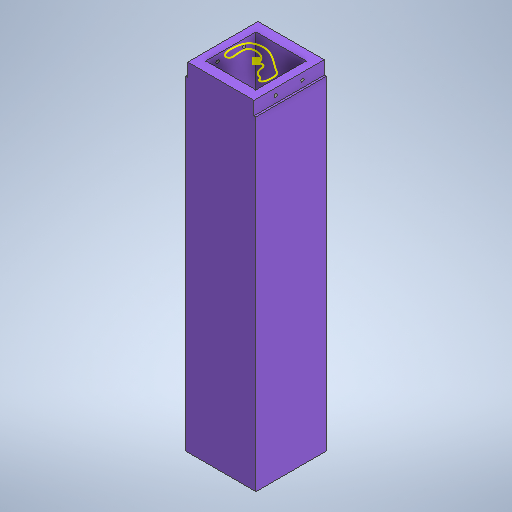
# Autodesk Inventor part: TS_Magazin_int
Saved by Autodesk Inventor 2025.2 (Build 292293000, 293)
## iProperties
Created: 2025-05-27
Part Number: TS_Magazin_int
Material: Generisch
Document SubType Name: Modeling
Designer: tino
Density: 1 g/cm^3
Appearance: Vorgabe
Mass: 3200 g
Surface Area: 1728 cm^2
Volume: 3200 cm^3
Author: tino
Autodesk Inventor part; units mm, degrees
ref_plane "YZ Plane" through (0, 0, 0) normal (1, 0, 0) x (0, 1, 0)
ref_plane "XZ Plane" through (0, 0, 0) normal (0, 1, 0) x (-1, 0, 0)
ref_plane "XY Plane" through (0, 0, 0) normal (0, 0, 1) x (1, 0, 0)
sketch "Skizze1" plane through (0, 0, 0) normal (0, 0, 1) x (1, 0, 0)
  line L0 (-52.5, 52.5) -> (52.5, 52.5)
  line L1 (52.5, 52.5) -> (52.5, -52.5)
  line L2 (52.5, -52.5) -> (-52.5, -52.5)
  line L3 (-52.5, -52.5) -> (-52.5, 52.5)
  line L4 (-52.5, 52.5) -> (52.5, -52.5) construction
  line L5 (52.5, 52.5) -> (-52.5, -52.5) construction
  point P0 (0, 0)
  dimension "d0" = 105
  dimension "d1" = 105
  constraints: 12 end point, 2 midpoint, 2 parallel, 1 horizontal, 1 perpendicular
  measures "d0" distance of L0.start L0.end
  measures "d1" distance of L0.end L1.end
extrude "Extrusion1" add sketch "Skizze1" along normal blind 505
sketch "Skizze2" plane through (0, 0, 505) normal (0, 0, 1) x (1, 0, 0)
  spline S0 degree 3 poles (30.8941, -22.3608) (33.2455, -20.1357) (33.4278, -16.4642) (34.1009, -12.3897) (34.4408, -6.5615) (32.3239, 0.3889) (27.6464, 2.563) (18.7777, 8.3579) (6.0522, 19.3643) (-10.5838, 24.0919) (-22.9306, 22.7109) (-28.1368, 17.5955) (-28.9312, 16.6042) knots 0 0 0 0 0.05535 0.076528 0.211782 0.295547 0.382964 0.432922 0.754884 0.81234 0.967238 1 1 1 1
  spline S1 degree 3 poles (-28.9312, 16.6042) (-32.363, 12.3217) (-33.922, 4.96) (-34.2212, -5.2183) (-33.7128, -11.7973) (-30.1787, -16.4552) (-26.4199, -18.3019) (-21.7499, -13.8164) (-22.8916, -9.4321) (-23.5075, -1.7153) (-24.1566, 7.4044) (-16.6489, 14.0721) (-3.6681, 12.4997) (3.1986, 4.5284) (3.2907, 1.6248) (4.5253, 0.0908) (6.4773, -0.7371) (8.3789, 1.0013) (13.1845, -1.004) (13.6371, -9.218) (17.043, -16.25) (23.1831, -17.8066) (25.3482, -18.6226) (26.133, -19.8789) (26.5745, -22.0211) (27.7048, -23.641) (30.0236, -23.1574) (30.8172, -22.4336) (30.8941, -22.3608) knots 0 0 0 0 0.14153 0.17035 0.245987 0.25892 0.290227 0.326265 0.372233 0.38898 0.482096 0.508256 0.624416 0.647418 0.715274 0.72607 0.746892 0.801722 0.811885 0.848514 0.916356 0.943374 0.948219 0.962959 0.96651 0.98188 0.998188 1 1 1 1
  arc A0 (27.4787, -6.7498) -> (23.9934, -5.2356) centre (25, -7.687) ccw
  line L0 (27.4787, -6.7498) -> (26.0066, -10.1384)
  arc A1 (22.5213, -8.6242) -> (26.0066, -10.1384) centre (25, -7.687) ccw
  line L1 (22.5213, -8.6242) -> (23.9934, -5.2356)
  line L2 (22.5213, -8.6242) -> (23.9934, -5.2356)
  arc A2 (22.5213, -8.6242) -> (26.0066, -10.1384) centre (25, -7.687) ccw
  line L3 (27.4787, -6.7498) -> (26.0066, -10.1384)
  arc A3 (27.4787, -6.7498) -> (23.9934, -5.2356) centre (25, -7.687) ccw
  line L4 (-52.5, 52.5) -> (-52.5, -52.5) construction
  line L5 (-52.5, 0) -> (52.5, 0) construction
  line L6 (52.5, -52.5) -> (52.5, 52.5) construction
  line L7 (-34.1215, 23.4036) -> (-34.1215, -17.2518) construction
  line L8 (34.1216, 27.1841) -> (34.1216, -29.8621) construction
  line L9 (-36.6715, 23.259) -> (37.4151, 23.259) construction
  line L10 (-34.1215, -23.2592) -> (37.4151, -23.2592) construction
  point P0 (0, 0)
  point P1 (0, 0)
  dimension "d4" = 34.1215
  dimension "d6" = 34.1216
  dimension "d10" = 23.259
  dimension "d11" = 23.2592
  constraints: 18 end point, 8 point on circle, 4 centre point, 4 vertical, 3 midpoint, 2 horizontal, 2 perpendicular, 4 other
  measures "d4" distance from line of L7 point (0, 0)
  measures "d6" distance from line of L8 point (0, 0)
  measures "d10" distance from line of point (0, 0) L9
  measures "d11" distance from line of point (0, 0) L10
extrude "Extrusion2" cut sketch "Skizze2" against normal blind 505 contours S1 S0 | L0 A1 L1 A0
sketch "Skizze4" plane through (0, 0, 505) normal (0, 0, 1) x (1, 0, 0)
  point P0 (0, 0)
  constraints: 2 other
sketch "Skizze5" plane through (0, 0, 505) normal (0, 0, 1) x (1, 0, 0)
  line L0 (-37.5, 37.5) -> (37.5, 37.5)
  line L1 (37.5, 37.5) -> (37.5, -37.5)
  line L2 (37.5, -37.5) -> (-37.5, -37.5)
  line L3 (-37.5, -37.5) -> (-37.5, 37.5)
  line L4 (-37.5, 37.5) -> (37.5, -37.5) construction
  line L5 (37.5, 37.5) -> (-37.5, -37.5) construction
  spline S0 degree 3 poles (-28.9312, 16.6042) (-28.1368, 17.5955) (-22.9306, 22.7109) (-10.5838, 24.0919) (6.0522, 19.3643) (18.7777, 8.3579) (27.6464, 2.563) (32.3239, 0.3889) (34.4408, -6.5615) (34.1009, -12.3897) (33.4278, -16.4642) (33.2455, -20.1357) (30.8941, -22.3608) knots 0 0 0 0 0.032762 0.18766 0.245116 0.567078 0.617036 0.704453 0.788218 0.923472 0.94465 1 1 1 1
  spline S1 degree 3 poles (30.8941, -22.3608) (30.8172, -22.4336) (30.0236, -23.1574) (27.7048, -23.641) (26.5745, -22.0211) (26.133, -19.8789) (25.3482, -18.6226) (23.1831, -17.8066) (17.043, -16.25) (13.6371, -9.218) (13.1845, -1.004) (8.3789, 1.0013) (6.4773, -0.7371) (4.5253, 0.0908) (3.2907, 1.6248) (3.1986, 4.5284) (-3.6681, 12.4997) (-16.6489, 14.0721) (-24.1566, 7.4044) (-23.5075, -1.7153) (-22.8916, -9.4321) (-21.7499, -13.8164) (-26.4199, -18.3019) (-30.1787, -16.4552) (-33.7128, -11.7973) (-34.2212, -5.2183) (-33.922, 4.96) (-32.363, 12.3217) (-28.9312, 16.6042) knots 0 0 0 0 0.001812 0.01812 0.03349 0.037041 0.051781 0.056626 0.083644 0.151486 0.188115 0.198278 0.253108 0.27393 0.284726 0.352582 0.375584 0.491744 0.517904 0.61102 0.627767 0.673735 0.709773 0.74108 0.754013 0.82965 0.85847 1 1 1 1
  point P0 (0, 0)
  dimension "d18" = 75
  dimension "d19" = 75
  constraints: 12 end point, 2 midpoint, 2 parallel, 1 horizontal, 1 perpendicular
  measures "d18" distance of L0.start L0.end
  measures "d19" distance of L0.end L1.end
extrude "Extrusion3" cut sketch "Skizze5" against normal blind 505
sketch "Skizze8" plane through (52.5, -52.5, 0) normal (1, 0, 0) x (0, 0, -1)
  line L0 (-505, 0) -> (-505, 105) projected
  line L1 (0, 105) -> (-505, 105) projected
  line L2 (-505, 0) -> (-485, 0)
  line L3 (-485, 0) -> (-485, 105)
  line L4 (-485, 105) -> (-505, 105)
  line L5 (-505, 105) -> (-505, 0)
  point P0 (0, 52.5)
  dimension "d33" = 20
  constraints: 8 end point, 2 parallel, 1 horizontal, 1 perpendicular, 1 point on line
  measures "d33" distance between parallel lines of L0 L3
extrude "Extrusion5" cut sketch "Skizze8" against normal blind 3
mirror "Spiegeln2" about plane through (0, 0, 0) normal (1, 0, 0) of "Extrusion5"
sketch "Skizze9" plane through (49.5, -52.5, 0) normal (1, 0, 0) x (0, 0, -1)
  line L0 (-505, 0) -> (-505, 105) projected
  line L1 (-505, 105) -> (-485, 105) projected
  point P0 (0, 52.5)
  point P1 (-495, 32.5)
  point P2 (-495, 72.5)
  dimension "d36" = 10
  dimension "d37" = 40
  dimension "d38" = 32.5
  constraints: 1 vertical alignment
  measures "d36" distance from line of L0 point (-495, 72.5)
  measures "d37" distance of point (-495, 72.5) point (-495, 32.5)
  measures "d38" distance from line of L1 point (-495, 72.5)
hole "Bohrung2" at (49.5, -20, 495) at (49.5, 20, 495) direction (-1, 0, 0) diameter 4.917 depth 12 tip angle 118 thread size "M6x1" class "6H" standard "ISO Metric profile"
mirror "Spiegeln3" about plane through (0, 0, 0) normal (1, 0, 0) of "Bohrung2"
sketch "Skizze11" plane through (0, 0, 0) normal (0, 0, -1) x (-1, 0, 0)
  line L0 (52.5, 52.5) -> (52.5, -52.5) projected
  line L1 (52.5, -52.5) -> (-52.5, -52.5) projected
  point P0 (0, 0)
  point P1 (45, -45)
  dimension "d46" = 7.5
  dimension "d47" = 7.5
  measures "d46" distance from line of point (45, -45) L0
  measures "d47" distance from line of point (45, -45) L1
hole "Bohrung3" at (-45, -45, 0) direction (0, 0, 1) diameter 4.917 depth 14 tip angle 118 thread size "M6x1" class "6H" standard "ISO Metric profile"
pattern_circular "Runde Anordnung1" count 4 over 360 about axis through (0, 0, -10) along (0, 0, 1) of "Bohrung3"
equation "\"d0\" = Magazin_Laenge"
equation "\"d1\" = Magazin_Breite"
equation "\"d2\" = Magazin_Hoehe"
equation "\"d12\" = Magazin_Hoehe"
equation "\"d18\" = Magazin_Breite - 2 * Wanddicke"
equation "\"d19\" = Magazin_Laenge - 2 * Wanddicke"
equation "\"d20\" = Magazin_Hoehe"
equation "\"d33\" = oberer_Absatz"
equation "\"d36\" = Bohrungsversatz_oben"
equation "\"d37\" = Bohrungsabstand_oben"
equation "\"d38\" = 0.5 * Magazin_Breite - 0.5 * Bohrungsabstand_oben"
equation "\"d46\" = 0.5 * Wanddicke"
equation "\"d47\" = d46"
equation "\"Magazin_Hoehe\" = 505"
equation "\"Magazin_Laenge\" = Magazin_Breite"
equation "\"Wanddicke\" = 15"
equation "\"Bohrungsversatz_oben\" = 10"
equation "\"Bohrungsabstand_oben\" = 40"
equation "\"oberer_Absatz\" = 20"
equation "\"Magazin_Breite\" = 105"
